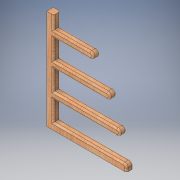
# Autodesk Inventor part: snowboard rack
Saved by Autodesk Inventor 2016 (Build 200138000, 138)
## iProperties
Created: 2017-02-05
Part Number: snowboard rack
Material: Wood (Birch)
Document SubType Name: Modeling
Designer: jwillauer
Density: 0.55 g/cm^3
Appearance: Birch - Natural Polished
Author: jwillauer
Autodesk Inventor part; units mm, degrees
ref_plane "YZ Plane" through (0, 0, 0) normal (1, 0, 0) x (0, 1, 0)
ref_plane "XZ Plane" through (0, 0, 0) normal (0, 1, 0) x (-1, 0, 0)
ref_plane "XY Plane" through (0, 0, 0) normal (0, 0, 1) x (1, 0, 0)
sketch "Sketch1" plane through (0, 0, 0) normal (0, 0, 1) x (1, 0, 0)
  line L0 (-190.2533, 169.37) -> (-164.8533, 169.37)
  line L1 (114.5467, -186.23) -> (114.5467, -211.63)
  line L2 (114.5467, -211.63) -> (-190.2533, -211.63)
  line L3 (-190.2533, -211.63) -> (-190.2533, 169.37)
  line L4 (114.5467, -186.23) -> (-164.8533, -186.23)
  line L5 (-164.8533, -186.23) -> (-164.8533, -110.03)
  line L6 (-164.8533, -110.03) -> (89.1467, -110.03)
  line L7 (89.1467, -84.63) -> (-164.8533, -84.63)
  line L8 (-164.8533, -84.63) -> (-164.8533, -8.43)
  line L9 (-164.8533, -8.43) -> (51.0467, -8.43)
  line L10 (51.0467, -8.43) -> (51.0467, 16.97)
  line L11 (51.0467, 16.97) -> (-164.8533, 16.97)
  line L12 (-164.8533, 16.97) -> (-164.8533, 93.17)
  line L13 (-164.8533, 93.17) -> (-12.4533, 93.17)
  line L14 (-12.4533, 93.17) -> (-12.4533, 118.57)
  line L15 (-12.4533, 118.57) -> (-164.8533, 118.57)
  line L16 (-164.8533, 118.57) -> (-164.8533, 169.37)
  line L17 (89.1467, -84.63) -> (89.1467, -110.03)
  point P0 (0, 0)
  dimension "d0" = 381
  dimension "d1" = 304.8
  dimension "d2" = 25.4
  dimension "d3" = 25.4
  dimension "d5" = 25.4
  dimension "d6" = 25.4
  dimension "d7" = 25.4
  dimension "d8" = 76.2
  dimension "d9" = 76.2
  dimension "d10" = 76.2
  dimension "d11" = 152.4
  dimension "d12" = 215.9
  dimension "d13" = 254
  constraints: 36 end point, 8 perpendicular, 5 point on line, 2 horizontal, 2 parallel, 2 vertical
  measures "d0" distance of L2.end L0.start
  measures "d1" distance of L1.end L2.end
  measures "d2" distance between parallel lines of L3 L12
  measures "d3" distance between parallel lines of L2 L4
  measures "d5" distance between parallel lines of L7 L6
  measures "d6" distance between parallel lines of L11 L9
  measures "d7" distance between parallel lines of L15 L13
  measures "d8" distance between parallel lines of L6 L4
  measures "d9" distance between parallel lines of L9 L7
  measures "d10" distance between parallel lines of L13 L11
  measures "d11" distance of L14.end L15.end
  measures "d12" distance of L10.end L11.end
  measures "d13" distance of L7.start L7.end
extrude "Extrusion1" add sketch "Sketch1" along normal blind 25.4
fillet "Fillet1" radius 12.7 5 edges at (114.5467, -186.23, 12.7) (89.1467, -84.63, 12.7) (89.1467, -110.03, 12.7) (51.0467, 16.97, 12.7) (51.0467, -8.43, 12.7)
fillet "Fillet1" radius 12.7 2 edges at (-12.4533, 118.57, 12.7) (-12.4533, 93.17, 12.7)
fillet "Fillet2" radius 6.35 10 edges at (-16.1731, 114.8502, 25.4) (-12.4533, 105.87, 25.4) (-16.1731, 96.8897, 25.4) (-95.0033, 93.17, 25.4) (-95.0033, 118.57, 25.4) (-16.1731, 114.8502, 0) (-12.4533, 105.87, 0) (-16.1731, 96.8897, 0) (-95.0033, 93.17, 0) (-95.0033, 118.57, 0)
fillet "Fillet3" radius 6.35 38 edges at (-164.8533, 115.395, 25.4) (-164.8533, 143.97, 25.4) (-164.8533, 115.395, 0) (-164.8533, 143.97, 0) (-164.8533, 96.345, 25.4) (-164.8533, 55.07, 25.4) (-164.8533, 96.345, 0) (-164.8533, 55.07, 0) (47.3269, 13.2502, 25.4) (51.0467, 4.27, 25.4) (47.3269, -4.7103, 25.4) (-63.2533, -8.43, 25.4) (-63.2533, 16.97, 25.4) (47.3269, 13.2502, 0) (51.0467, 4.27, 0) (47.3269, -4.7103, 0) (-63.2533, -8.43, 0) (-63.2533, 16.97, 0) (-164.8533, -46.53, 25.4) (-164.8533, -46.53, 0) (85.4269, -106.3103, 25.4) (89.1467, -97.33, 25.4) (85.4269, -88.3498, 25.4) (-44.2033, -84.63, 25.4) (-44.2033, -110.03, 25.4) (85.4269, -106.3103, 0) (89.1467, -97.33, 0) (85.4269, -88.3498, 0) (-44.2033, -110.03, 0) (-44.2033, -84.63, 0) (-164.8533, -148.13, 25.4) (-164.8533, -148.13, 0) (110.8269, -189.9498, 25.4) (114.5467, -205.28, 25.4) (-31.5033, -186.23, 25.4) (110.8269, -189.9498, 0) (114.5467, -205.28, 0) (-31.5033, -186.23, 0)
body "Solid1"
